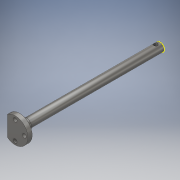
# Autodesk Inventor part: slide rod
Saved by Autodesk Inventor 2017 (Build 210142000, 142)
## iProperties
Created: 2016-12-06
Part Number: slide rod
Material: Stainless Steel, 440C
Document SubType Name: Modeling
Designer: qupec
Density: 7.75 g/cm^3
Appearance: Semi-Polished
Mass: 18.0788 g
Surface Area: 15.3279 cm^2
Volume: 2.33275 cm^3
Author: qupec
Autodesk Inventor part; units mm, degrees
ref_plane "YZ Plane" through (0, 0, 0) normal (1, 0, 0) x (0, 1, 0)
ref_plane "XY Plane" through (0, 0, 0) normal (0, 0, 1) x (1, 0, 0)
sketch "Sketch1" plane through (0, 0, 0) normal (0, 0, 1) x (1, 0, 0)
  circle A0 centre (0, 0) radius 3.175
  dimension "d0" = 6.35
  constraints: 1 centre point, 1 coincident
  measures "d0" diameter of A0
extrude "Extrusion1" add sketch "Sketch1" along normal mid plane 106.045
sketch "Sketch2" plane through (0, 0, 53.0225) normal (0, 0, 1) x (1, 0, 0)
  point P0 (0, 0)
  point P1 (0, 0)
  constraints: 1 coincident
sketch "Sketch3" plane through (0, 0, -53.0225) normal (0, 0, -1) x (-1, 0, 0)
  point P0 (0, 0)
  point P1 (0, 0)
  constraints: 1 coincident
sketch "Sketch4" plane through (0, 0, -53.0225) normal (0, 0, -1) x (-1, 0, 0)
  circle A0 centre (0, 0) radius 1.651
  dimension "d3" = 3.302
  constraints: 1 centre point, 1 coincident
  measures "d3" diameter of A0
extrude "Extrusion2" [suppressed]
thread "Thread1" size "6-32 UNC" class "2B" standard "ANSI Unified Screw Threads" full length
ref_plane "Work Plane1" through (0, 3.175, 0) normal (0, 1, 0) x (-1, 0, 0)
sketch "Sketch5" plane through (0, 3.175, 0) normal (0, 1, 0) x (-1, 0, 0)
  circle A0 centre (0, -49.8475) radius 1.4224
  line L0 (-3.175, -53.0225) -> (3.175, -53.0225) projected
  point P0 (0, 0)
  dimension "d8" = 2.8448
  dimension "d9" = 3.175
  constraints: 1 centre point
  measures "d8" diameter of A0
  measures "d9" distance from line of L0 A0.centre
extrude "Extrusion3" cut sketch "Sketch5" against normal through all
thread "Thread3" size "4-40 UNC" class "2B" standard "ANSI Unified Screw Threads" full length
sketch "Sketch7" plane through (0, 0, 0) normal (1, 0, 0) x (0, 1, 0)
  line L0 (3.175, 53.0225) -> (-3.175, 53.0225) projected
  line L1 (3.175, -53.0225) -> (3.175, 53.0225) projected
  line L2 (-3.175, -53.0225) -> (-3.175, 53.0225) projected
  line L3 (3.175, 53.0225) -> (15.875, 53.0225)
  line L4 (3.175, 53.0225) -> (-3.175, 53.0225) projected
  line L5 (0, 53.0225) -> (0, 40.8931) construction
  line L6 (15.875, 53.0225) -> (15.875, 49.8475)
  line L7 (15.875, 49.8475) -> (6.35, 49.8475)
  line L8 (6.35, 49.8475) -> (3.175, 40.3225)
  line L9 (3.175, 40.3225) -> (3.175, 53.0225)
  point P0 (0, 0)
  dimension "d17" = 12.7
  dimension "d18" = 9.525
  dimension "d20" = 3.175
  dimension "d21" = 12.7
  constraints: 12 end point, 2 vertical, 1 collinear, 1 horizontal, 1 midpoint, 1 perpendicular, 1 point on line
  measures "d17" distance of L1.end L3.end
  measures "d18" distance of L6.end L7.end
  measures "d20" distance of L3.end L6.end
  measures "d21" distance of L1.end L8.end
revolve "Revolution1" [suppressed]
fillet "Fillet1" [suppressed]
fillet "Fillet2" [suppressed]
sketch "Sketch8" plane through (0, 0, 45.4025) normal (0, 0, -1) x (-1, 0, 0)
  circle A0 centre (0, 0) radius 15.875 projected
  circle A1 centre (0, 0) radius 8.6384 projected
  point P0 (0, 0)
  point P1 (-12.2567, 0)
  point P2 (-15.875, 0)
  point P3 (-8.6384, 0)
  dimension "d26" = 3.6183
  dimension "d28" = 7.2366
  constraints: 2 horizontal alignment, 2 other
  measures "d26" distance of point (-12.257, 0) point (-15.875, 0)
  measures "d28" distance of point (-15.875, 0) point (-8.638, 0)
hole "Hole1" [suppressed]
pattern_circular "Circular Pattern1" [suppressed]
sketch "Sketch9" plane through (0, 0, 53.0225) normal (0, 0, 1) x (1, 0, 0)
  line L0 (5.08, 12.7) -> (-5.08, 12.7)
  line L1 (-5.08, 12.7) -> (-5.08, -12.7)
  line L2 (-5.08, -12.7) -> (5.08, -12.7)
  line L3 (5.08, -12.7) -> (5.08, 12.7)
  circle A0 centre (0, 0) radius 3.175 projected
  line L4 (3.175, 1.0866) -> (3.175, -1.4346) construction
  dimension "d39" = 10.16
  dimension "d40" = 6.35
  dimension "d41" = 5.08
  dimension "d42" = 25.4
  dimension "d43" = 12.7
  dimension "d44" = 1.905
  constraints: 10 end point, 3 parallel, 1 horizontal, 1 perpendicular, 1 tangent, 1 vertical
  measures "d39" distance of L1.end L2.end
  measures "d40" diameter of A0
  measures "d41" distance from line of L3 point (0, 0)
  measures "d42" distance of L2.end L0.start
  measures "d43" distance from line of point (0, 0) L0
  measures "d44" distance between parallel lines of L3 L4
extrude "Extrusion4" [suppressed]
sketch "Sketch10" plane through (0, 0, 0) normal (1, 0, 0) x (0, 1, 0)
  line L0 (3.175, -53.0225) -> (3.175, 53.0225) projected
  line L1 (0, -80.01) -> (0, 80.01) projected
  line L2 (3.175, -53.0225) -> (3.175, 53.0225) projected
  line L3 (3.175, 53.0225) -> (-3.175, 53.0225) projected
  line L4 (4.191, 49.8475) -> (9.271, 49.8475)
  line L5 (9.271, 49.8475) -> (9.271, 53.0225)
  line L6 (9.271, 53.0225) -> (3.175, 53.0225)
  line L7 (3.175, 44.7675) -> (3.81, 44.7675)
  line L8 (3.81, 44.7675) -> (4.191, 49.8475)
  point P0 (0, 0)
  point P1 (3.175, 39.0525)
  dimension "d57" = 5.08
  dimension "d58" = 1.016
  dimension "d59" = 5.08
  dimension "d60" = 3.175
  dimension "d80" = 0.635
  constraints: 10 end point, 2 horizontal, 2 perpendicular, 2 point on line
  measures "d57" distance of L4.start L4.end
  measures "d58" distance from line of L0 L4.start
  measures "d59" vertical distance of L4.start L7.start
  measures "d60" distance between parallel lines of L6 L4
  measures "d80" distance of L7.start L7.end
revolve "Revolution2" add sketch "Sketch10" angle 360 about axis through (0, 0, -10) along (0, 0, 1)
sketch "Sketch12" plane through (0, 0, 49.8475) normal (0, 0, -1) x (-1, 0, 0)
  circle A0 centre (0, 0) radius 4.191 projected
  circle A1 centre (0, 0) radius 9.271 projected
  line L0 (0, 0) -> (-9.271, 0) construction
  point P0 (-6.731, 0)
  point P1 (-4.191, 0)
  dimension "d61" = 5.08
  dimension "d62" = 2.54
  dimension "d73" = 0
  dimension "d74" = 0
  constraints: 2 end point, 2 point on circle, 1 horizontal, 1 horizontal alignment, 1 other
  measures "d61" distance of A1.start point (-4.191, 0)
  measures "d62" distance of point (-6.731, 0) A1.start
  measures "d73" vertical distance of A1.start point (-4.191, 0)
  measures "d74" distance from line of L0 A1.start
hole "Hole2" at (6.731, 0, 49.8475) direction (0, 0, 1) diameter 2.8448 depth 25.4 tip angle 118
pattern_circular "Circular Pattern2" count 4 over 360 about axis through (0, 0, -10) along (0, 0, 1) of "Hole2" skipped copies 3
sketch "Sketch14" plane through (0, 0, 53.0225) normal (0, 0, 1) x (1, 0, 0)
  circle A0 centre (0, 0) radius 4.191 projected
  circle A1 centre (0, 0) radius 3.175 projected
  circle A2 centre (0, 0) radius 9.271 projected
  line L0 (-5.715, 7.3) -> (-5.715, -7.3)
  arc A3 (-5.715, 7.3) -> (-5.715, -7.3) centre (0, 0) ccw
  dimension "d79" = 5.715
  constraints: 4 point on circle, 2 end point, 1 centre point, 1 coincident, 1 concentric, 1 vertical
  measures "d79" distance from line of point (0, 0) L0
extrude "Extrusion6" cut sketch "Sketch14" against normal through all contours L0 A2 picked at (-6.9003, 0)
sketch "Sketch15" plane through (0, 0, -53.0225) normal (0, 0, -1) x (-1, 0, 0)
  circle A0 centre (0, 0) radius 3.175 projected
equation "\"d26\" = 0.5 * d28"
equation "\"d41\" = 0.5 * d39"
equation "\"d43\" = 0.5 * d42"
equation "\"d62\" = 0.5 * d61"
equation "\"d34\" = d26"
body "Solid1"
